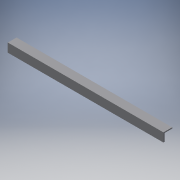
# Autodesk Inventor part: 15102898-16-P-0219
Saved by Autodesk Inventor 2017 (Build 210142000, 142)
## iProperties
Created: 2016-10-10
Part Number: 15102898-16-P-0219
Material: Generic
Document SubType Name: Modeling
Designer: gus
Density: 1 g/cm^3
Appearance: Default
Author: gus
Autodesk Inventor part; units mm, degrees
ref_plane "YZ Plane" through (0, 0, 0) normal (1, 0, 0) x (0, 1, 0)
ref_plane "XZ Plane" through (0, 0, 0) normal (0, 1, 0) x (-1, 0, 0)
ref_plane "XY Plane" through (0, 0, 0) normal (0, 0, 1) x (1, 0, 0)
sketch "Sketch1" plane through (0, 0, 0) normal (1, 0, 0) x (0, 1, 0)
  line L0 (0, 0) -> (25.4, 0)
  line L1 (25.4, 0) -> (25.4, -25.4)
  line L2 (22.225, -25.4) -> (22.225, -3.175)
  line L3 (22.225, -3.175) -> (0, -3.175)
  line L4 (0, 0) -> (0, -3.175)
  line L5 (22.225, -25.4) -> (25.4, -25.4)
  dimension "d1" = 25.4
  dimension "d2" = 3.175
  dimension "d5" = 25.4
  dimension "d6" = 22.225
  constraints: 12 end point, 2 perpendicular, 1 horizontal, 1 vertical, 1 other
  measures "d1" distance of L0.end L1.end
  measures "d2" distance between parallel lines of L1 L2
  measures "d5" distance of L0.start L0.end
  measures "d6" distance of L2.start L2.end
ref_plane "Work Plane1" through (121.4904, -591.0492, 62.9788) normal (-1, 0, 0) x (0, -0.0011424, 0.9999993)
ref_plane "Work Plane2" through (594.413, -591.0492, 62.9788) normal (1, 0, 0) x (0, 0.9999993, 0.0011424)
ref_plane "Work Plane3" through (121.4904, -685.829, -0.8415) normal (-1, 0, 0) x (0, 0, 1)
ref_plane "Work Plane4" through (572.188, -685.8218, 2.3335) normal (1, 0, 0) x (0, 1, 0)
ref_plane "Work Plane5" through (571.4614, -9.58, -1.5962) normal (1, 0, 0) x (0, 1, 0)
ref_plane "Work Plane6" through (98.5388, -9.58, -1.5962) normal (-1, 0, 0) x (0, 0, 1)
extrude "Extrusion1" add sketch "Sketch1" against normal up to surface (472.9226 mm away) from surface at 571.4614
body "Solid1"
